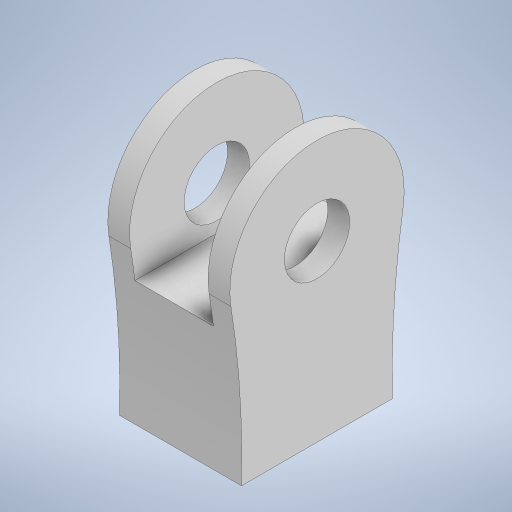
# Autodesk Inventor part: cabeza_obj1
Saved by Autodesk Inventor 2023.2 (Build 272271030, 271C)
## iProperties
Created: 2023-02-25
Part Number: cabeza_obj1
Material: Generic
Document SubType Name: Modeling
Designer: Cris Pat
Density: 1 g/cm^3
Appearance: Default
Author: Cris Pat
Autodesk Inventor part; units mm, degrees
ref_plane "YZ Plane" through (0, 0, 0) normal (1, 0, 0) x (0, 1, 0)
ref_plane "XZ Plane" through (0, 0, 0) normal (0, 1, 0) x (-1, 0, 0)
ref_plane "XY Plane" through (0, 0, 0) normal (0, 0, 1) x (1, 0, 0)
sketch "Sketch1" plane through (0, 0, 0) normal (1, 0, 0) x (0, 1, 0)
  circle A0 centre (0, 0) radius 7.5
  arc A1 (-3.1515, -19.7501) -> (-3.1515, 19.7501) centre (0, 0) ccw
  circle A2 centre (-34.667, -217.2515) radius 200 construction
  line L0 (-10, 17.3205) -> (-10, -17.3205) construction
  line L1 (-40, 17.3226) -> (-40, -17.3226) construction
  line L2 (0, 0) -> (-40, 0) construction
  circle A3 centre (-34.667, 217.2515) radius 200 construction
  line L3 (-40, 17.3226) -> (-40, -17.3226)
  arc A4 (-40, 17.3226) -> (-3.1515, 19.7501) centre (-34.667, 217.2515) ccw
  arc A5 (-3.1515, -19.7501) -> (-40, -17.3226) centre (-34.667, -217.2515) ccw
  dimension "d6" = 15
  dimension "d7" = 40
  dimension "d8" = 400
  dimension "d9" = 34.667
  dimension "d10" = 10
  dimension "d11" = 30
  constraints: 10 point on circle, 8 end point, 6 centre point, 3 coincident, 2 concentric, 2 vertical, 1 collinear, 1 midpoint, 1 perpendicular, 1 symmetric about line, 1 tangent, 1 other
  measures "d6" diameter of A0
  measures "d7" diameter of A1
  measures "d8" diameter of A2
  measures "d9" horizontal distance of A2.centre A0.centre
  measures "d10" distance from line of L0 A0.centre
  measures "d11" distance between parallel lines of L1 L0
extrude "Extrusion1" add sketch "Sketch1" along normal mid plane 28
sketch "Sketch3" plane through (0, 0, 0) normal (0, 0, 1) x (1, 0, 0)
  line L0 (-14, 20) -> (14, 20) construction
  line L1 (-14, -3.1515) -> (14, -3.1515) construction
  line L2 (14, -40) -> (14, -3.1515) construction
  line L3 (14, -40) -> (-14, -40) construction
  line L4 (-14, -3.1515) -> (-14, -40) construction
  line L5 (-9, 20) -> (9, 20)
  line L6 (9, 20) -> (9, -10)
  line L7 (9, -10) -> (-9, -10)
  line L8 (-9, -10) -> (-9, 20)
  point P0 (0, 0)
  point P1 (0, 20)
  point P2 (0, 20)
  dimension "d19" = 18
  dimension "d21" = 10
  constraints: 8 end point, 2 midpoint, 2 parallel, 1 coincident, 1 horizontal, 1 horizontal alignment, 1 perpendicular
  measures "d19" distance of L6.end L7.end
  measures "d21" distance from line of point (0, 0) L7
extrude "Extrusion3" cut sketch "Sketch3" along normal through all both and the other way through all
sketch "Sketch4" plane through (-9, -10, -18.7784) normal (0, 1, 0) x (1, 0, 0)
  line L0 (23, -1.4559) -> (-5, -1.4559) construction
  line L1 (23, -36.101) -> (23, -1.4559) construction
  line L2 (-5, -36.101) -> (23, -36.101) construction
  line L3 (-5, -1.4559) -> (-5, -36.101) construction
  line L4 (-5, -36.101) -> (23, -36.101) construction
  line L5 (9, -36.101) -> (9, -1.4559) construction
  line L6 (-5, -1.4559) -> (-5, -36.101) construction
  line L7 (-5, -18.7784) -> (23, -18.7784) construction
  line L8 (23, -36.101) -> (23, -1.4559) construction
  circle A0 centre (9, -18.7784) radius 4.3
  circle A1 centre (9, -18.7784) radius 2.75
  point P0 (9, -18.7784)
  dimension "d24" = 8.6
  dimension "d25" = 5.5
  constraints: 6 midpoint, 4 end point, 2 centre point, 1 coincident
  measures "d24" diameter of A0
  measures "d25" diameter of A1
extrude "Extrusion4" cut sketch "Sketch4" against normal blind 3.3 contours A0 | A1
extrude "Extrusion5" cut sketch "Sketch4" against normal through all contours A1
body "Solid1"
